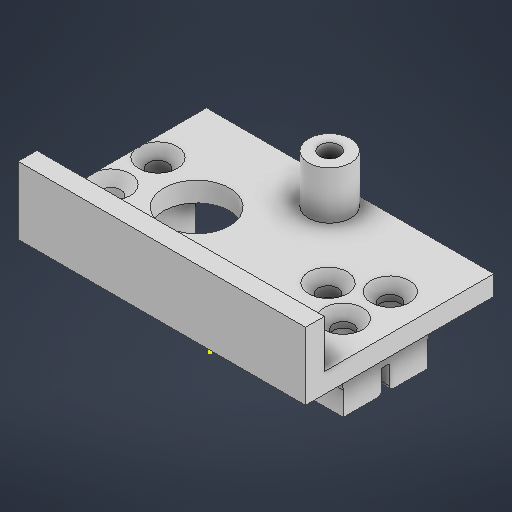
# Autodesk Inventor part: ПЕРЕДНИЙ ЗАХВАТ
Saved by Autodesk Inventor 2025 (Build 290162000, 162)
## iProperties
Created: 2025-02-17
Part Number: ПЕРЕДНИЙ ЗАХВАТ
Material: Типовые
Document SubType Name: Modeling
Designer: Phantom
Density: 1 g/cm^3
Appearance: По умолчанию
Author: Phantom
Autodesk Inventor part; units mm, degrees
ref_plane "YZ Plane" through (0, 0, 0) normal (1, 0, 0) x (0, 1, 0)
ref_plane "XZ Plane" through (0, 0, 0) normal (0, 1, 0) x (-1, 0, 0)
ref_plane "XY Plane" through (0, 0, 0) normal (0, 0, 1) x (1, 0, 0)
sketch "Эскиз1" plane through (0, 0, 0) normal (0, 1, 0) x (-1, 0, 0)
  line L0 (-30, 30.5) -> (30, 30.5)
  line L1 (30, 30.5) -> (30, -30.5)
  line L2 (30, -30.5) -> (-30, -30.5)
  line L3 (-30, -30.5) -> (-30, 30.5)
  line L4 (-30, 30.5) -> (30, 30.5) construction
  circle A0 centre (0, -25.5) radius 2.1
  circle A1 centre (-14, -11.15) radius 2.1
  circle A2 centre (14, -11.15) radius 7
  point P0 (0, 0)
  dimension "d0" = 60
  dimension "d2" = 61
  dimension "d3" = 30
  dimension "d4" = 4.2
  dimension "d5" = 5
  dimension "d6" = 4.2
  dimension "d7" = 19.35
  dimension "d8" = 28
  dimension "d9" = 14
  dimension "d11" = 19.35
  dimension "d13" = 16
  constraints: 10 end point, 3 centre point, 2 horizontal, 2 parallel, 1 collinear, 1 perpendicular
  measures "d0" distance of L0.start L0.end
  measures "d2" distance of L0.end L1.end
  measures "d3" distance from line of L3 A0.centre
  measures "d4" diameter of A0
  measures "d5" distance from line of L2 A0.centre
  measures "d6" diameter of A1
  measures "d7" distance from line of L2 A1.centre
  measures "d8" distance of A1.centre A2.centre
  measures "d9" diameter of A2
  measures "d11" distance from line of L2 A2.centre
  measures "d13" distance from line of L3 A1.centre
extrude "Выдавливание1" add sketch "Эскиз1" along normal blind 3.2
sketch "Эскиз2" plane through (0, 3.2, 0) normal (0, 1, 0) x (1, 0, 0)
  line L0 (30, 30.5) -> (-30, 30.5) projected
  line L1 (-30, 30.5) -> (-30, -5.65)
  line L2 (-30, 30.5) -> (-30, -30.5) projected
  line L3 (-30, -5.65) -> (30, -5.65)
  line L4 (-30, -5.65) -> (30, -5.65)
  line L5 (30, -5.65) -> (30, -9.65)
  line L6 (30, -9.65) -> (-30, -9.65)
  line L7 (-30, -9.65) -> (-30, -5.65)
  circle A0 centre (0, 25.5) radius 2.1 projected
  circle A1 centre (0, 25.5) radius 4.5
  point P0 (0, 0)
  dimension "d16" = 36.15
  dimension "d17" = 60
  dimension "d18" = 4
  dimension "d19" = 9
  constraints: 12 end point, 2 parallel, 2 perpendicular, 1 centre point, 1 coincident, 1 horizontal, 1 point on line
  measures "d16" distance of L0.end L1.end
  measures "d17" distance of L5.end L6.end
  measures "d18" distance of L4.end L5.end
  measures "d19" diameter of A1
extrude "Выдавливание2" add sketch "Эскиз2" along normal blind 10.2
sketch "Эскиз3" plane through (0, 0, 0) normal (0, -1, 0) x (1, 0, 0)
  arc A0 (-23.25, -20.65) -> (-22.25, -21.65) centre (-22.25, -20.65) ccw
  line L0 (-23.25, -20.65) -> (-23.25, -1.65)
  arc A1 (-22.25, -0.65) -> (-23.25, -1.65) centre (-22.25, -1.65) ccw
  line L1 (17.25, -0.65) -> (-22.25, -0.65)
  arc A2 (18.25, -1.65) -> (17.25, -0.65) centre (17.25, -1.65) ccw
  line L2 (18.25, -20.65) -> (18.25, -1.65)
  arc A3 (17.25, -21.65) -> (18.25, -20.65) centre (17.25, -20.65) ccw
  line L3 (17.25, -21.65) -> (-22.25, -21.65)
  circle A4 centre (-27.25, -16.15) radius 2.1
  circle A5 centre (-27.25, -6.15) radius 2.1
  circle A6 centre (22.25, -6.15) radius 2.1
  circle A7 centre (22.25, -16.15) radius 2.1
  line L4 (2.4, 0.15) -> (9.6, 0.15)
  circle A8 centre (-14, -11.15) radius 7 projected
  line L5 (-27.25, -2.15) -> (-23.25, -2.15)
  line L6 (-27.25, -2.15) -> (-31.25, -2.15)
  line L7 (-31.25, -2.15) -> (-31.25, -20.15)
  line L8 (-31.25, -20.15) -> (-23.25, -20.15)
  line L9 (-2.5, -0.65) -> (-2.5, -38)
  line L10 (18.25, -20.65) -> (18.25, -1.65)
  circle A9 centre (22.25, -16.15) radius 2.1
  circle A10 centre (22.25, -6.15) radius 2.1
  line L11 (22.25, -2.15) -> (18.25, -2.15)
  line L12 (22.25, -2.15) -> (26.25, -2.15)
  line L13 (26.25, -2.15) -> (26.25, -20.15)
  line L14 (26.25, -20.15) -> (18.25, -20.15)
  point P0 (0, 0)
  point P1 (-14, -11.15)
  point P2 (26, -11.15)
  constraints: 30 end point, 10 centre point, 8 point on circle, 7 symmetric about line, 6 point on line, 2 perpendicular, 2 vertical, 1 coincident, 1 midpoint, 2 other
extrude "Выдавливание3" add sketch "Эскиз3" along normal blind 11 contours L8 L7 L6 L5 L0 | L2 L11 L12 L13 L14
sketch "Эскиз4" plane through (0, 0, 0) normal (0, 1, 0) x (1, 0, 0)
  line L0 (-30, 20.15) -> (-30, 2.15) projected
  line L1 (-31.25, 20.15) -> (-30, 20.15) projected
  line L2 (-31.25, 2.15) -> (-31.25, 20.15) projected
  line L3 (-30, 2.15) -> (-31.25, 2.15) projected
  line L4 (30, -9.65) -> (-30, -9.65) projected
  line L5 (-30, -9.65) -> (-30, -30.5) projected
  line L6 (-30, -30.5) -> (30, -30.5) projected
  line L7 (30, -30.5) -> (30, -9.65) projected
  line L8 (-30, -30.5) -> (-31.25, -30.5)
  line L9 (-31.25, -30.5) -> (-31.25, 30.5)
  line L10 (-31.25, 30.5) -> (-30, 30.5)
  line L11 (-30, 30.5) -> (-30, -30.5)
  line L12 (30, 30.5) -> (-30, 30.5) projected
  point P0 (0, 0)
  dimension "d25" = 0
  constraints: 8 end point, 2 parallel, 1 collinear, 1 horizontal, 1 perpendicular
  measures "d25" distance between parallel lines of L10 L12
extrude "Выдавливание4" add sketch "Эскиз4" along normal up to surface (3.2 mm away) contours L0 L3 L2 L1 | L1 L9 L10 L11 | L11 L5 L8 L9 L3
sketch "Эскиз5" plane through (0, 3.2, 0) normal (0, 1, 0) x (1, 0, 0)
  circle A0 centre (14, 11.15) radius 2.1 projected
  circle A1 centre (-14, 11.15) radius 7 projected
  circle A2 centre (0, 25.5) radius 4.5 projected
  line L0 (30, -9.65) -> (-30, -9.65) projected
  line L1 (-30, -5.65) -> (-30, -9.65) projected
  line L2 (-30, -5.65) -> (30, -5.65) projected
  line L3 (30, -5.65) -> (30, 30.5) projected
  line L4 (30, 30.5) -> (-31.25, 30.5) projected
  line L5 (-31.25, -30.5) -> (-31.25, 30.5) projected
  line L6 (30, -30.5) -> (-31.25, -30.5) projected
  line L7 (30, -30.5) -> (30, -9.65) projected
  line L8 (-30, -9.65) -> (-31.25, -9.65)
  line L9 (-31.25, -9.65) -> (-31.25, -5.65)
  line L10 (-31.25, -5.65) -> (-30, -5.65)
  line L11 (-30, -5.65) -> (-30, -9.65)
  point P0 (0, 0)
  constraints: 8 end point, 2 parallel, 1 horizontal, 1 perpendicular, 1 point on line
extrude "Выдавливание5" add sketch "Эскиз5" along normal up to surface (10.2 mm away) contours L8 L5 L10 L1
sketch "Эскиз6" plane through (0, -11, 0) normal (0, -1, 0) x (1, 0, 0)
  point P0 (0, 0)
sketch "Эскиз7" plane through (0, -11, 0) normal (0, -1, 0) x (1, 0, 0)
  line L0 (18.25, -20.15) -> (18.25, -2.15) projected
  line L1 (18.25, -11.15) -> (26.25, -11.15)
  line L2 (26.25, -2.15) -> (26.25, -20.15) projected
  line L3 (18.25, -10.4) -> (26.25, -10.4)
  line L4 (26.25, -10.4) -> (26.25, -11.9)
  line L5 (26.25, -11.9) -> (18.25, -11.9)
  line L6 (18.25, -11.9) -> (18.25, -10.4)
  line L7 (18.25, -10.4) -> (26.25, -11.9) construction
  line L8 (26.25, -10.4) -> (18.25, -11.9) construction
  line L9 (-31.25, -20.15) -> (-23.25, -20.15) projected
  line L10 (18.25, -20.15) -> (-23.25, -20.15)
  line L11 (-2.5, -20.15) -> (-2.5, 5)
  line L12 (-23.25, -11.15) -> (-31.25, -11.15)
  line L13 (-23.25, -10.4) -> (-31.25, -10.4)
  line L14 (-31.25, -10.4) -> (-31.25, -11.9)
  line L15 (-31.25, -11.9) -> (-23.25, -11.9)
  line L16 (-23.25, -11.9) -> (-23.25, -10.4)
  line L17 (-23.25, -10.4) -> (-31.25, -11.9) construction
  line L18 (-31.25, -10.4) -> (-23.25, -11.9) construction
  point P0 (0, 0)
  point P1 (22.25, -11.15)
  point P2 (-27.25, -11.15)
  dimension "d30" = 8
  dimension "d31" = 1.5
  constraints: 32 end point, 7 symmetric about line, 6 midpoint, 2 horizontal, 2 parallel, 1 perpendicular, 1 vertical
  measures "d30" distance of L4.end L5.end
  measures "d31" distance of L3.end L4.end
extrude "Выдавливание6" cut sketch "Эскиз7" against normal blind 5
fillet "Сопряжение1" radius 1 4 edges at (22.25, -11, -11.9) (22.25, -11, -10.4) (-27.25, -11, -11.9) (-27.25, -11, -10.4)
sketch "Эскиз8" plane through (0, -11, 0) normal (0, -1, 0) x (1, 0, 0)
  circle A0 centre (-27.25, -6.15) radius 2.1 projected
  circle A1 centre (-27.25, -16.15) radius 2.1 projected
  circle A2 centre (22.25, -6.15) radius 2.1 projected
  circle A3 centre (22.25, -16.15) radius 2.1 projected
  point P0 (0, 0)
extrude "Выдавливание7" cut sketch "Эскиз8" against normal through all
sketch "Эскиз9" plane through (0, 3.2, 0) normal (0, 1, 0) x (1, 0, 0)
  line L0 (30, -9.65) -> (-31.25, -9.65) projected
  line L1 (-31.25, -30.5) -> (-31.25, -9.65) projected
  line L2 (30, -30.5) -> (-31.25, -30.5) projected
  line L3 (30, -30.5) -> (30, -9.65) projected
  point P0 (0, 0)
extrude "Выдавливание8" cut sketch "Эскиз9" against normal blind 10
chamfer "Фаска1" distance 2 angle 45 5 edges at (16.1, 3.2, -11.15) (20.15, 3.2, -16.15) (20.15, 3.2, -6.15) (-29.35, 3.2, -6.15) (-29.35, 3.2, -16.15)
sketch "Эскиз10" plane through (0, 0, 0) normal (0, -1, 0) x (1, 0, 0)
  circle A0 centre (-14, -11.15) radius 7 projected
  circle A1 centre (14, -11.15) radius 2.1 projected
  circle A2 centre (0, -25.5) radius 2.1 projected
  line L0 (30, 9.65) -> (-31.25, 9.65) projected
  line L1 (-31.25, -30.5) -> (-31.25, -20.15) projected
  line L2 (-23.25, -2.15) -> (-23.25, -20.15) projected
  line L3 (-31.25, -2.15) -> (-31.25, 9.65) projected
  line L4 (30, -30.5) -> (-31.25, -30.5) projected
  line L5 (30, 9.65) -> (30, -30.5) projected
  line L6 (18.25, -20.15) -> (18.25, -2.15) projected
  line L7 (26.25, -2.15) -> (26.25, -20.15) projected
  line L8 (-23.25, -2.15) -> (-23.25, 2.85) projected
  line L9 (-23.25, 2.85) -> (-31.25, 2.85) projected
  line L10 (-31.25, 2.85) -> (-31.25, -2.15) projected
  line L11 (-31.25, -2.15) -> (-23.25, -2.15) projected
  line L12 (-23.25, -25.15) -> (-23.25, -20.15) projected
  line L13 (-23.25, -20.15) -> (-31.25, -20.15) projected
  line L14 (-31.25, -20.15) -> (-31.25, -25.15) projected
  line L15 (-31.25, -25.15) -> (-23.25, -25.15) projected
  line L16 (26.25, -25.15) -> (26.25, -20.15) projected
  line L17 (26.25, -20.15) -> (18.25, -20.15) projected
  line L18 (18.25, -20.15) -> (18.25, -25.15) projected
  line L19 (18.25, -25.15) -> (26.25, -25.15) projected
  line L20 (18.25, 2.85) -> (18.25, -2.15) projected
  line L21 (18.25, -2.15) -> (26.25, -2.15) projected
  line L22 (26.25, -2.15) -> (26.25, 2.85) projected
  line L23 (26.25, 2.85) -> (18.25, 2.85) projected
  line L24 (26.25, -20.15) -> (18.25, -20.15) projected
  line L25 (18.25, -2.15) -> (26.25, -2.15) projected
  line L26 (-31.25, -2.15) -> (-23.25, -2.15) projected
  line L27 (-31.25, -20.15) -> (-23.25, -20.15) projected
  point P0 (0, 0)
extrude "Выдавливание9" add sketch "Эскиз10" along normal blind 1 contours L5 L4 L1 L15 L12 L2 L8 L9 L3 L0 | L9 L8 L11 L3 | L1 L13 L12 L15 | L6 L21 L7 L17 | L17 L16 L19 L18 | L20 L23 L22 L21
fillet "Сопряжение3" radius 5 4 edges at (-27.25, -1, -20.15) (-27.25, -1, -2.15) (22.25, -1, -20.15) (22.25, -1, -2.15)
